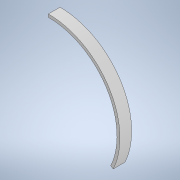
# Autodesk Inventor part: printTest120degeePortion
Saved by Autodesk Inventor 2021 (Build 250183000, 183)
## iProperties
Created: 2020-07-16
Part Number: printTest120degeePortion
Material: Generic
Document SubType Name: Modeling
Designer: robst
Density: 1 g/cm^3
Appearance: Default
Author: robst
Autodesk Inventor part; units mm, degrees
ref_plane "YZ Plane" through (0, 0, 0) normal (1, 0, 0) x (0, 1, 0)
ref_plane "XZ Plane" through (0, 0, 0) normal (0, 1, 0) x (-1, 0, 0)
ref_plane "XY Plane" through (0, 0, 0) normal (0, 0, 1) x (1, 0, 0)
sketch "Sketch1" plane through (0, 0, 0) normal (0, 0, 1) x (1, 0, 0)
  arc A0 (135.5385, -62.4294) -> (0, 149.225) centre (0, 0) ccw
  arc A1 (141.0601, -65.6173) -> (0, 155.575) centre (0, 0) ccw
  line L0 (0, 149.225) -> (0, 155.575)
  line L1 (135.5385, -62.4294) -> (141.0601, -65.6173)
  dimension "d0" = 298.45
  dimension "d1" = 311.15
  dimension "d2" = 120
  constraints: 4 end point, 4 point on circle, 2 centre point, 2 coincident, 1 vertical
  measures "d0" diameter of A0
  measures "d1" diameter of A1
  measures "d2" angle of L1 L0
extrude "Extrusion1" add sketch "Sketch1" along normal mid plane 25.4
body "Solid1"
